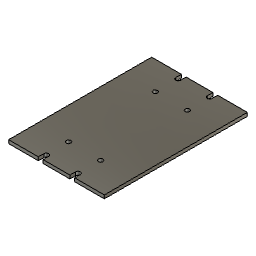
well_catridge_working_electrode_water_cut (Autodesk Fusion 360 design; units mm, degrees)
Autodesk Fusion 360 part; units mm, degrees
note: some values were not read from the file. Set by a fixed rule: which sketch regions a step uses.
sketch "Sketch1" plane through (0, 0, 0) normal (0, 0, 1) x (1, 0, 0)
  line L0 (-42.5, 63.5) -> (-42.5, -63.5)
  line L1 (42.5, -63.5) -> (42.5, 63.5)
  line L2 (42.5, 63.5) -> (-42.5, -63.5) construction
  line L3 (-42.5, 63.5) -> (42.5, -63.5) construction
  line L4 (-42.5, 63.5) -> (-32.5, 63.5) construction
  line L5 (-80, 0) -> (75, 0) construction
  line L6 (0, 85) -> (0, -82.7869) construction
  line L7 (14.25, 38.5) -> (-14.25, 38.5) construction
  line L8 (-14.25, 38.5) -> (-14.25, -38.5) construction
  line L9 (-14.25, -38.5) -> (14.25, -38.5) construction
  line L10 (14.25, -38.5) -> (14.25, 38.5) construction
  line L11 (14.25, 38.5) -> (-14.25, -38.5) construction
  line L12 (-14.25, 38.5) -> (14.25, -38.5) construction
  circle A0 centre (14.25, 38.5) radius 2
  circle A1 centre (-14.25, 38.5) radius 2
  circle A2 centre (-14.25, -38.5) radius 2
  circle A3 centre (14.25, -38.5) radius 2
  line L13 (0, -63.5) -> (11.9, -63.5) construction
  line L14 (0, -63.5) -> (0, -58.5) construction
  line L15 (0, -58.5) -> (14, -58.5) construction
  line L16 (11.9, -63.5) -> (11.9, -58.5)
  line L17 (16.1, -58.5) -> (16.1, -63.5)
  arc A4 (16.1, -58.5) -> (11.9, -58.5) centre (14, -58.5) ccw
  line L18 (16.1, -63.5) -> (42.5, -63.5)
  line L19 (-11.9, -63.5) -> (-11.9, -58.5)
  arc A5 (-11.9, -58.5) -> (-16.1, -58.5) centre (-14, -58.5) ccw
  line L20 (-16.1, -58.5) -> (-16.1, -63.5)
  line L21 (-11.9, 63.5) -> (-11.9, 58.5)
  arc A6 (-16.1, 58.5) -> (-11.9, 58.5) centre (-14, 58.5) ccw
  line L22 (-16.1, 58.5) -> (-16.1, 63.5)
  line L23 (11.9, 63.5) -> (11.9, 58.5)
  arc A7 (11.9, 58.5) -> (16.1, 58.5) centre (14, 58.5) ccw
  line L24 (16.1, 58.5) -> (16.1, 63.5)
  line L25 (-42.5, -63.5) -> (-16.1, -63.5)
  line L26 (-11.9, -63.5) -> (11.9, -63.5)
  line L27 (-16.1, 63.5) -> (-42.5, 63.5)
  line L28 (42.5, 63.5) -> (16.1, 63.5)
  line L29 (11.9, 63.5) -> (-11.9, 63.5)
  dimension "d1" = 85
  dimension "d2" = 127
  dimension "d12" = 28.5
  dimension "d13" = 77
  dimension "d14" = 4
  dimension "d15" = 4
  dimension "d16" = 4
  dimension "d17" = 4
  dimension "d18" = 11.9
  dimension "d19" = 5
  dimension "d20" = 14
  dimension "d21" = 4.2
  dimension "d22" = 5
  dimension "d23" = 5
  constraint horizontal L28
  constraint perpendicular L0 L28
  constraint parallel L25 L28
  constraint parallel L0 L1
  constraint perpendicular L0 L4
  constraint perpendicular L1 L5
  constraint perpendicular L6 L25
  constraint horizontal L7
  constraint perpendicular L7 L8
  constraint parallel L7 L9
  constraint parallel L8 L10
  constraint coincident L11 origin
  constraint coincident L12 origin
  constraint coincident L7.start L10.end
  constraint coincident L7.end L8.start
  constraint coincident L8.end L9.start
  constraint coincident L9.end L10.start
  constraint perpendicular L6 L13
  constraint perpendicular L14 L25
  constraint perpendicular L6 L15
  constraint coincident L15.end A4.centre
  constraint vertical L16
  constraint vertical L17
  constraint collinear L18 L25
  constraint coincident L13.start L25
  constraint symmetric L6 L13.end L19.start
  constraint symmetric L6 L16.end L19.end
  constraint symmetric L6 L17.start A5.end
  constraint symmetric L6 L17.end L20.end
  constraint symmetric L6 A4 A5
  constraint symmetric L5 L13.end L23.start
  constraint symmetric L5 L16.end L23.end
  constraint symmetric L5 L17.start A7.end
  constraint symmetric L5 L17.end L24.end
  constraint symmetric L5 A4 A7
  constraint symmetric L5 L19.start L21.start
  constraint symmetric L5 L19.end L21.end
  constraint symmetric L5 A5.end A6.start
  constraint symmetric L5 A5 A6
  constraint symmetric L5 L20.end L22.end
  constraint collinear L25 L26
  constraint collinear L27 L28
  constraint collinear L28 L29
  measures "d1" distance of L0.end L1.start
  measures "d2" distance of L0.start L0.end
  measures "d12" distance of L8.end L9.end
  measures "d13" distance of L7.end L8.end
  measures "d14" diameter of A0
  measures "d15" diameter of A1
  measures "d16" diameter of A2
  measures "d17" diameter of A3
  measures "d18" distance of L13.start L13.end
  measures "d19" distance of L13.start L14.end
  measures "d20" distance of L14.end L15.end
  measures "d21" diameter of A4
  measures "d22" distance of L13.end L16.end
  measures "d23" distance of L17.start L17.end
extrude "Extrude1" add sketch "Sketch1" along normal blind 3
